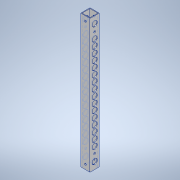
# Autodesk Inventor part: ロボットベース15x15_2
Saved by Autodesk Inventor 2020.3 (Build 243373000, 373)
## iProperties
Created: 2020-07-04
Part Number: ロボットベース15x15_2
Material: アルミニウム 6061
Document SubType Name: Modeling
Designer: totot
Density: 2.7 g/cm^3
Appearance: アルミニウム - フラット
Author: totot
Autodesk Inventor part; units mm, degrees
ref_plane "YZ Plane" through (0, 0, 0) normal (1, 0, 0) x (0, 1, 0)
ref_plane "XZ Plane" through (0, 0, 0) normal (0, 1, 0) x (-1, 0, 0)
ref_plane "XY Plane" through (0, 0, 0) normal (0, 0, 1) x (1, 0, 0)
sketch "スケッチ1" plane through (0, 0, 0) normal (0, 1, 0) x (-1, 0, 0)
  line L0 (0, 0) -> (-15, 0)
  line L1 (-15, 0) -> (-15, 15)
  line L2 (-15, 15) -> (0, 15)
  line L3 (0, 15) -> (0, 0)
  line L4 (-1.2, 13.8) -> (-13.8, 13.8)
  line L5 (-13.8, 13.8) -> (-13.8, 1.2)
  line L6 (-13.8, 1.2) -> (-1.2, 1.2)
  line L7 (-1.2, 1.2) -> (-1.2, 13.8)
  dimension "d0" = 15
  dimension "d1" = 15
  dimension "d2" = 1.2
  dimension "d3" = 1.2
  dimension "d4" = 1.2
  dimension "d5" = 1.2
  constraints: 16 end point, 4 parallel, 2 horizontal, 2 perpendicular
  measures "d0" distance of L1.end L2.end
  measures "d1" distance of L0.end L1.end
  measures "d2" distance between parallel lines of L2 L4
  measures "d3" distance between parallel lines of L7 L3
  measures "d4" distance between parallel lines of L1 L5
  measures "d5" distance between parallel lines of L0 L6
extrude "押し出し1" add sketch "スケッチ1" along normal blind 215
sketch "スケッチ2" plane through (0, 0, 15) normal (0, 0, 1) x (1, 0, 0)
  line L0 (0, 0) -> (0, 215) projected
  line L1 (0, 0) -> (15, 0) projected
  line L2 (0, 215) -> (15, 215) projected
  point P0 (7.5, 7.5)
  point P1 (7.5, 207.5)
  dimension "d8" = 7.5
  dimension "d9" = 7.5
  dimension "d10" = 7.5
  dimension "d11" = 7.5
  measures "d8" distance from line of point (7.5, 7.5) L0
  measures "d9" distance from line of point (7.5, 207.5) L0
  measures "d10" distance from line of point (7.5, 7.5) L1
  measures "d11" distance from line of point (7.5, 207.5) L2
hole "穴1" at (7.5, 7.5, 15) at (7.5, 207.5, 15) direction (0, 0, -1) diameter 3 end through all
sketch "スケッチ3" plane through (0, 0, 0) normal (-1, 0, 0) x (0, 0, 1)
  line L0 (0, 0) -> (0, 215) projected
  line L1 (0, 0) -> (15, 0) projected
  line L2 (0, 215) -> (15, 215) projected
  point P0 (7.5, 22.5)
  point P1 (7.5, 192.5)
  dimension "d19" = 7.5
  dimension "d20" = 7.5
  dimension "d21" = 22.5
  dimension "d22" = 22.5
  measures "d19" distance from line of point (7.5, 22.5) L0
  measures "d20" distance from line of point (7.5, 192.5) L0
  measures "d21" distance from line of point (7.5, 22.5) L1
  measures "d22" distance from line of point (7.5, 192.5) L2
hole "穴2" at (0, 22.5, 7.5) at (0, 192.5, 7.5) direction (1, 0, 0) diameter 3 end through all
sketch "スケッチ4" plane through (15, 0, 15) normal (1, 0, 0) x (0, 0, -1)
  line L0 (0, 0) -> (15, 0) projected
  circle A0 centre (7.5, 22.5) radius 1.5 projected
  line L1 (15, 0) -> (15, 215) projected
  line L2 (0, 215) -> (15, 215) projected
  circle A1 centre (7.5, 192.5) radius 1.5 projected
  point P0 (7.5, 11.25)
  point P1 (7.5, 203.75)
  point P2 (7.5, 182.5)
  point P3 (7.5, 172.5)
  point P4 (7.5, 162.5)
  point P5 (7.5, 152.5)
  point P6 (7.5, 142.5)
  point P7 (7.5, 132.5)
  point P8 (7.5, 122.5)
  point P9 (7.5, 112.5)
  point P10 (7.5, 102.5)
  point P11 (7.5, 92.5)
  point P12 (7.5, 82.5)
  point P13 (7.5, 72.5)
  point P14 (7.5, 62.5)
  point P15 (7.5, 52.5)
  point P16 (7.5, 42.5)
  point P17 (7.5, 32.5)
  dimension "d30" = 22.5
  dimension "d31" = 11.25
  dimension "d32" = 7.5
  dimension "d33" = 11.25
  dimension "d34" = 7.5
  dimension "d35" = 170
  dimension "d36" = 7.5
  dimension "d37" = 10
  dimension "d40" = 10
  constraints: 1 vertical, 15 other
  measures "d30" distance from line of L0 A0.centre
  measures "d31" distance of point (7.5, 11.25) A0.centre
  measures "d32" distance from line of point (7.5, 11.25) L1
  measures "d33" distance from line of L2 point (7.5, 203.75)
  measures "d34" distance from line of point (7.5, 203.75) L1
  measures "d35" distance of A1.centre A0.centre
  measures "d36" distance from line of point (7.5, 182.5) L1
  measures "d37" distance of point (7.5, 182.5) A1.centre
  measures "d40" distance of point (7.5, 182.5) point (7.5, 172.5)
hole "穴3" at (15, 11.25, 7.5) at (15, 203.75, 7.5) at (15, 182.5, 7.5) at (15, 172.5, 7.5) at (15, 162.5, 7.5) at (15, 152.5, 7.5) at (15, 142.5, 7.5) at (15, 132.5, 7.5) at (15, 122.5, 7.5) at (15, 112.5, 7.5) at (15, 102.5, 7.5) at (15, 92.5, 7.5) at (15, 82.5, 7.5) at (15, 72.5, 7.5) at (15, 62.5, 7.5) at (15, 52.5, 7.5) at (15, 42.5, 7.5) at (15, 32.5, 7.5) direction (-1, 0, 0) diameter 8.5 end through all
equation "\"d3\" = d2"
equation "\"d4\" = d3"
equation "\"d5\" = d2"
equation "\"d9\" = d8"
equation "\"d10\" = d8"
equation "\"d11\" = d9"
equation "\"d20\" = d19"
equation "\"d22\" = d21"
equation "\"d31\" = 0.5 * d30"
equation "\"d33\" = d31"
